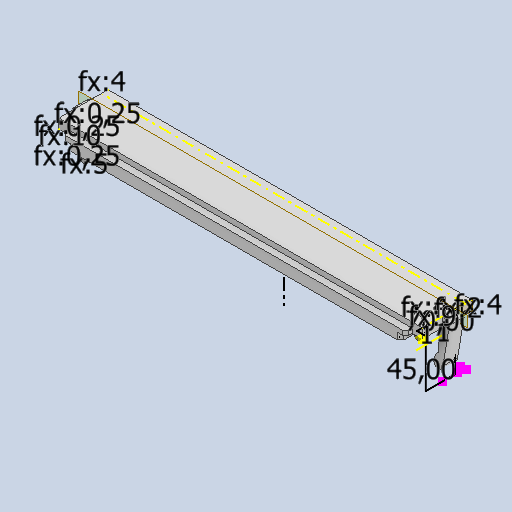
# Autodesk Inventor part: Generischer Gehäuse Deckel
Saved by Autodesk Inventor 2025.2 (Build 292293000, 293)
## iProperties
Created: 2025-11-01
Part Number: Generischer Gehäuse Deckel
Material: Generisch
Document SubType Name: Modeling
Designer: leowa
Density: 1 g/cm^3
Appearance: Vorgabe
Author: leowa
Autodesk Inventor part; units mm, degrees
ref_plane "YZ Plane" through (0, 0, 0) normal (1, 0, 0) x (0, 1, 0)
ref_plane "XZ Plane" through (0, 0, 0) normal (0, 1, 0) x (-1, 0, 0)
ref_plane "XY Plane" through (0, 0, 0) normal (0, 0, 1) x (1, 0, 0)
sketch "Skizze1" plane through (0, 0, 0) normal (0, 1, 0) x (-1, 0, 0)
  line L0 (0, 0) -> (108, 0)
  line L1 (108, 0) -> (108, -15)
  line L2 (108, -15) -> (0, -15)
  line L3 (0, -15) -> (0, 0)
  dimension "d0" = 108
  dimension "d1" = 15
  constraints: 8 end point, 2 parallel, 1 horizontal, 1 perpendicular
  measures "d0" distance of L1.end L2.end
  measures "d1" distance of L2.end L0.start
extrude "Extrusion1" add sketch "Skizze1" along normal blind 3
sketch "Skizze2" plane through (0, 0, 0) normal (0, -1, 0) x (1, 0, 0)
  line L0 (-108, 0) -> (0, 0) projected
  line L1 (-106.35, 0) -> (-1.65, 0)
  line L2 (-1.65, 0) -> (-1.65, 2)
  line L3 (-1.65, 2) -> (-106.35, 2)
  line L4 (-106.35, 2) -> (-106.35, 0)
  line L5 (-108, -15) -> (-108, 0) projected
  line L6 (0, -15) -> (-108, -15) projected
  line L7 (-54, -15) -> (-54, 78)
  point P0 (-54, 0)
  point P1 (-54, 2)
  dimension "d4" = 1.65
  dimension "d5" = 2
  constraints: 10 end point, 2 parallel, 1 horizontal, 1 midpoint, 1 perpendicular, 1 point on line, 1 vertical, 1 other
  measures "d4" distance between parallel lines of L4 L5
  measures "d5" distance between parallel lines of L0 L3
extrude "Extrusion2" add sketch "Skizze2" against normal blind 1.35 contours L4 L3 L7 L0 | L7 L3 L2 L0
sketch "Skizze3" plane through (0, 0, 0) normal (0, -1, 0) x (1, 0, 0)
  line L0 (0, -15) -> (-108, -15) projected
  line L1 (-106.65, -15) -> (-1.35, -15)
  line L2 (-1.35, -15) -> (-1.35, -13)
  line L3 (-1.35, -13) -> (-106.65, -13)
  line L4 (-106.65, -13) -> (-106.65, -15)
  line L5 (-54, -15) -> (-54, 54)
  line L6 (-108, -15) -> (-108, 0) projected
  point P0 (0, 0)
  dimension "d8" = 1.35
  dimension "d9" = 2
  constraints: 10 end point, 2 parallel, 1 horizontal, 1 midpoint, 1 perpendicular, 1 point on line, 1 vertical, 1 other
  measures "d8" distance between parallel lines of L6 L4
  measures "d9" distance of L3.end L1.start
extrude "Extrusion3" cut sketch "Skizze3" against normal blind 1.65
ref_plane "Arbeitsebene1" through (0, 3, -10) normal (0, 0, -1) x (-1, 0, 0)
sketch "Skizze4" plane through (0, 0, 0) normal (0, -1, 0) x (1, 0, 0)
  line L0 (21.6, -10) -> (-129.6, -10) projected
  line L1 (-104.875, -10) -> (-3.125, -10)
  line L2 (-3.125, -10) -> (-3.125, -13)
  line L3 (-3.125, -13) -> (-104.875, -13)
  line L4 (-104.875, -13) -> (-104.875, -10)
  line L5 (-106.65, -13) -> (-1.35, -13) projected
  line L6 (-1.35, -13) -> (-1.35, -15) projected
  line L7 (0, -15) -> (-108, -15) projected
  line L8 (-54, -15) -> (-54, 34)
  point P0 (0, 0)
  point P1 (-3.125, -10)
  dimension "d36" = 101.75
  constraints: 10 end point, 2 parallel, 1 collinear, 1 horizontal, 1 midpoint, 1 perpendicular, 1 point on line, 1 vertical, 1 other
  measures "d36" distance of L2.end L3.end
extrude "Extrusion4" add sketch "Skizze4" along normal blind 2 contours L2 L3 L8 L0 | L8 L3 L4 L0
sketch "Skizze5" plane through (0, 0, 0) normal (0, -1, 0) x (1, 0, 0)
  line L0 (-3.125, -8.02) -> (-104.875, -8.02)
  line L1 (-104.875, -8.02) -> (-104.875, 2)
  line L2 (-104.875, 2) -> (-3.125, 2)
  line L3 (-3.125, 2) -> (-3.125, -8.02)
  line L4 (-3.125, -10) -> (-104.875, -10) projected
  line L5 (-104.875, -10) -> (-104.875, -13) projected
  line L6 (-3.125, -13) -> (-3.125, -10) projected
  line L7 (-1.65, 2) -> (-106.35, 2) projected
  point P0 (0, 0)
  dimension "d16" = 1.98
  constraints: 8 end point, 3 collinear, 2 parallel, 1 horizontal, 1 perpendicular
  measures "d16" distance between parallel lines of L4 L0
extrude "Extrusion5" add sketch "Skizze5" along normal up to surface (2 mm away)
sketch "Skizze6" plane through (-108, 0, -15) normal (-1, 0, 0) x (0, 0, 1)
  line L0 (15, 3) -> (0, 3) projected
  line L1 (0, 3) -> (15, 3)
  line L2 (15, 3) -> (15, 0)
  line L3 (15, 0) -> (0, 0)
  line L4 (0, 0) -> (0, 3)
  constraints: 8 end point, 2 parallel, 1 horizontal, 1 perpendicular
extrude "Extrusion6" add sketch "Skizze6" along normal blind 1.5
sketch "Skizze9" plane through (0, 0, 0) normal (1, 0, 0) x (0, 0, -1)
  line L0 (0, 0) -> (15, 0) projected
  line L1 (15, 0) -> (15, 3) projected
  line L2 (0, 3) -> (15, 3) projected
  line L3 (0, 0) -> (0, 3) projected
extrude "Extrusion9" add sketch "Skizze9" along normal blind 1.5
sketch "Skizze7" plane through (-109.5, 0, -15) normal (-1, 0, 0) x (0, 0, 1)
  line L0 (15, 0) -> (0, 0) projected
  line L1 (4, 0) -> (9, 0) construction
  line L2 (9, 0) -> (9, -10) construction
  line L3 (9, -10) -> (4, -10) construction
  line L4 (4, -10) -> (4, 0) construction
  line L5 (0, 3) -> (0, 0) projected
  line L6 (4.25, 0) -> (8.75, 0)
  line L7 (8.75, 0) -> (8.75, -10.25)
  line L8 (8.75, -10.25) -> (4.25, -10.25)
  line L9 (4.25, -10.25) -> (4.25, 0)
  point P0 (9, 0)
  point P1 (8.75, 0)
  point P2 (4.25, 0)
  dimension "d22" = 4
  dimension "d23" = 5
  dimension "d24" = 10
  dimension "d37" = 0.25
  dimension "d38" = 0.25
  dimension "d39" = 0.25
  constraints: 16 end point, 4 parallel, 2 horizontal, 2 perpendicular, 2 point on line
  measures "d22" distance between parallel lines of L4 L5
  measures "d23" distance of L2.end L3.end
  measures "d24" distance of L1.end L2.end
  measures "d37" distance between parallel lines of L4 L9
  measures "d38" distance between parallel lines of L2 L7
  measures "d39" distance between parallel lines of L3 L8
extrude "Extrusion7" add sketch "Skizze7" against normal blind 1.25
extrude "Extrusion11" add sketch "Skizze7" along normal blind 1.25 from surface at -111
sketch "Skizze8" plane through (-109.5, -10, -6.25) normal (0, 0, 1) x (1, 0, 0)
  line L0 (0, 13) -> (111, 13) projected
  line L1 (55.5, 13) -> (55.5, -32)
  line L2 (0, -0.25) -> (0, 10) projected
  line L3 (0, -0.25) -> (1.25, -0.25) projected
  line L4 (1.25, 10) -> (1.25, -0.25) projected
  line L5 (0, 10) -> (1.25, 10) projected
  line L6 (0, -0.25) -> (0, 10) projected
  line L7 (1.25, 10) -> (1.25, -0.25) projected
  line L8 (111, -0.25) -> (111, 10) projected
  arc A0 (2.75, -0.25) -> (1.25, 2.8725) centre (-1.25, -0.25) ccw
  arc A1 (0, -0.25) -> (2.75, -0.25) centre (1.375, -0.25) ccw
  line L9 (0, -0.25) -> (1.25, -0.25)
  line L10 (1.25, 2.8725) -> (0, 2.8725)
  line L11 (0, -0.25) -> (0, 2.8725)
  line L12 (111, -0.25) -> (109.75, -0.25)
  arc A2 (109.75, 2.8725) -> (108.25, -0.25) centre (112.25, -0.25) ccw
  arc A3 (108.25, -0.25) -> (111, -0.25) centre (109.625, -0.25) ccw
  line L13 (111, -0.25) -> (109.75, -0.25)
  line L14 (109.75, 2.8725) -> (111, 2.8725)
  line L15 (111, -0.25) -> (111, 2.8725)
  point P0 (1.25, -4.25)
  point P1 (0, 2.8725)
  dimension "d76" = 4
  dimension "d77" = 1.5
  constraints: 16 end point, 8 point on circle, 7 point on line, 7 symmetric about line, 4 centre point, 2 collinear, 2 tangent, 1 midpoint, 1 perpendicular, 1 vertical, 2 other
  measures "d76" radius of A0
  measures "d77" distance from line of A0.start L4
extrude "Extrusion8" add sketch "Skizze8" against normal up to surface (4.5 mm away) contours L2 L10 L4 L3 | L3 L4 A0 A1 | A3 A2 L14 L8
sketch "Skizze11" plane through (0.25, 0, -6.25) normal (0, 0, 1) x (1, 0, 0)
  line L0 (1.25, 3) -> (-109.75, 3) projected
  line L1 (-54.25, 3) -> (-54.25, -19)
  line L2 (-109.75, 3) -> (1.25, 3)
  arc A0 (-1.5, -10.25) -> (1.25, -10.25) centre (-0.125, -10.25) ccw projected
  line L3 (1.25, -10.25) -> (3.25, 1.5)
  line L4 (3.25, 1.5) -> (1.25, 3)
  line L5 (1.25, 3) -> (1.25, 0) projected
  line L6 (1.25, 1.5) -> (5.25, 1.5) construction
  line L7 (1.25, -10.25) -> (1.25, 3) construction
  line L8 (1.25, -10.25) -> (1.25, 0) construction
  line L9 (-109.75, -10.25) -> (-111.75, 1.5)
  line L10 (-111.75, 1.5) -> (-109.75, 3)
  line L11 (-109.75, 3) -> (-109.75, 0)
  line L12 (-109.75, -10.25) -> (-109.75, 3) construction
  line L13 (-109.75, -10.25) -> (-109.75, 0) construction
  line L14 (1.25, -10.25) -> (1.25, 3)
  line L15 (-109.75, 0) -> (-109.75, 3) projected
  line L16 (-109.75, -10.25) -> (-109.75, 3)
  point P0 (-109.75, 1.5)
  point P1 (-109.75, 0)
  point P2 (1.25, 0)
  dimension "d78" = 2
  constraints: 26 end point, 8 symmetric about line, 3 collinear, 3 midpoint, 1 horizontal, 1 vertical
  measures "d78" distance of L3.end L6.start
extrude "Extrusion12" add sketch "Skizze11" against normal up to surface (4.5 mm away)
sketch "Skizze12" plane through (-1.35, 1.65, -13) normal (0, 0, -1) x (-1, 0, 0)
  line L0 (1.775, -1.65) -> (1.775, -3.65) projected
  line L1 (1.775, -3.65) -> (3.2309, -7.65)
  line L2 (3.2309, -7.65) -> (4.2309, -7.65)
  line L3 (4.2309, -7.65) -> (5.6868, -3.65)
  line L4 (103.525, -3.65) -> (1.775, -3.65) projected
  line L5 (-1.6, -15.9) -> (-3.35, -15.9) projected
  line L6 (-2.85, 1.35) -> (108.15, 1.35) projected
  line L7 (52.65, 1.35) -> (52.65, -27)
  line L8 (1.775, -3.65) -> (5.6868, -3.65)
  line L9 (103.525, -3.65) -> (102.0691, -7.65)
  line L10 (102.0691, -7.65) -> (101.0691, -7.65)
  line L11 (101.0691, -7.65) -> (99.6132, -3.65)
  line L12 (103.525, -3.65) -> (99.6132, -3.65)
  point P0 (-1.35, -1.65)
  dimension "d52" = 70
  dimension "d53" = 1
  dimension "d55" = 4
  constraints: 18 end point, 3 symmetric about line, 1 collinear, 1 equal length, 1 midpoint, 1 perpendicular, 1 point on line, 1 vertical
  measures "d52" angle of L4 L1
  measures "d53" distance of L1.end L2.end
  measures "d55" distance between parallel lines of L4 L2
extrude "Extrusion13" add sketch "Skizze12" against normal up to surface (3 mm away)
extrude "Extrusion14" add sketch "Skizze12" against normal blind 3 from surface at -4.98
chamfer "Fasen2" distance 1 angle 45 4 edges at (-106.35, 0.675, 2) (-104.875, -1, 2) (-1.65, 0.675, 2) (-3.125, -1, 2)
ref_plane "Arbeitsebene2" through (1.5, 0, 0) normal (1, 0, 0) x (0, 0, -1)
sketch "Skizze13" plane through (1.5, 0, 0) normal (1, 0, 0) x (0, 0, -1)
  point P0 (0, 0)
sketch "Skizze14" plane through (1.5, 0, 0) normal (1, 0, 0) x (0, 0, -1)
  line L0 (-2, -2) -> (-1, -2) projected
  line L1 (-1, -2) -> (-2, -2) projected
  line L2 (5.02, -2) -> (-1, -2) projected
  line L3 (5.02, -2) -> (8.02, -2) projected
  line L4 (8.02, -2) -> (5.02, -2) projected
  line L5 (-1, -2) -> (5.02, -2) projected
  line L6 (10, -6) -> (10, -2) projected
  line L7 (10, -2) -> (10, -6) projected
  line L8 (10, 0) -> (10, -2) projected
  line L9 (10, 0) -> (10, -2) projected
  line L10 (10, -6) -> (10, -2) projected
  line L11 (10, -2) -> (10, -6) projected
  line L12 (0, 3) -> (6.25, 3) projected
  line L13 (6.25, 3) -> (0, 3) projected
  line L14 (10.75, 3) -> (6.25, 3) projected
  line L15 (15, 3) -> (10.75, 3) projected
  line L16 (10.75, 3) -> (15, 3) projected
  line L17 (6.25, 3) -> (10.75, 3) projected
  line L18 (10, -14.25) -> (1, -14.25)
  line L19 (1, -14.25) -> (1, 3)
  line L20 (1, 3) -> (10, 3)
  line L21 (10, 3) -> (10, -14.25)
  line L22 (10, 3) -> (12, 3)
  line L23 (12, 3) -> (12, -1)
  line L24 (12, -1) -> (10, -1)
  line L25 (10, -1) -> (10, 3)
  line L26 (1, 0.35) -> (-1.65, 3)
  line L27 (-1.65, 3) -> (1, 3)
  line L28 (-1, 1.35) -> (-2, 1.35) projected
  line L29 (-1, 1.35) -> (0, 1.35) projected
  line L30 (0, 1.35) -> (-1, 1.35) projected
  line L31 (-2, 1.35) -> (-1, 1.35) projected
  line L32 (0, 1.35) -> (1, 1.35) construction
  line L33 (6.25, -14.25) -> (10.75, -14.25) projected
  line L34 (6.25, -14.25) -> (10.75, -14.25) projected
  line L35 (6.25, -14.25) -> (10.75, -14.25) projected
  point P0 (0, 0)
  dimension "d64" = 9
  dimension "d65" = 2
  dimension "d66" = 4
  dimension "d67" = 45
  dimension "d69" = 1
  constraints: 22 end point, 4 parallel, 3 collinear, 3 horizontal, 3 perpendicular, 2 point on line
  measures "d64" distance between parallel lines of L19 L21
  measures "d65" distance of L23.end L24.end
  measures "d66" distance of L22.end L23.end
  measures "d67" angle of L19 L26
  measures "d69" distance of L26.start L32.end
equation "\"d0\" = Modul_Grundflächenlänge + 2 * Wandstärke"
equation "\"d1\" = Generische_Modulbreite"
equation "\"d2\" = Deckelstärke"
equation "\"d4\" = 0.55 * Basisstärke"
equation "\"d5\" = Modulüberlappung"
equation "\"d6\" = 0.45 * Deckelstärke"
equation "\"d8\" = 0.45 * Basisstärke"
equation "\"d9\" = Modulüberlappung"
equation "\"d10\" = 0.55 * Deckelstärke"
equation "\"d36\" = Modul_Grundflächenlänge - 0.5 * Stecktoleranz"
equation "\"d14\" = Deckel_Verstärkung"
equation "\"d16\" = 1.1 * Platinendicke"
equation "\"d20\" = Deckel_Klipperstärke"
equation "\"d31\" = Deckel_Klipperstärke"
equation "\"d22\" = Deckel_Klipperposition"
equation "\"d23\" = Deckel_Klippbreite"
equation "\"d24\" = Deckel_Klipplänge"
equation "\"d37\" = 0.5 * Stecktoleranz"
equation "\"d38\" = 0.5 * Stecktoleranz"
equation "\"d39\" = 0.5 * Stecktoleranz"
equation "\"d25\" = Deckel_Klipperstärke - 0.5 * Stecktoleranz"
equation "\"d40\" = Deckel_Klipperstärke - 0.5 * Stecktoleranz"
equation "\"d76\" = Deckelklipper_Radius"
equation "\"d77\" = Deckel_Klipptiefe"
equation "\"d55\" = Deckel_Einrastführungslänge"
equation "\"d64\" = Steckverbinder_Lochtiefe"
equation "\"d65\" = Steckverbinder_Absatzbreite"
equation "\"d66\" = Steckverbinder_Absatztiefe"
equation "\"Wandstärke\" = 3"
equation "\"Basisstärke\" = 3"
equation "\"Modulüberlappung\" = 2"
equation "\"Platinendicke\" = 1.8"
equation "\"Deckelstärke\" = 3"
equation "\"Seitenwand_Höhe\" = 39"
equation "\"Platinenposition\" = 5"
equation "\"d12\" = -Platinenposition"
equation "\"Deckel_Klippbreite\" = 5"
equation "\"Deckel_Klipplänge\" = 10"
equation "\"Deckel_Klipperposition\" = 4"
equation "\"Deckel_Klipperstärke\" = 1.5"
equation "\"Deckel_Klipptiefe\" = 1.5"
equation "\"Modul_Klipptiefe\" = 1.5"
equation "\"Modul_Klipperstärke\" = 1.5"
equation "\"Modul_Klipperposition\" = 7"
equation "\"Modul_Klipplänge\" = 8"
equation "\"Lüftungsraster\" = 2"
equation "\"Dings\" = 2"
equation "\"Modul_Grundflächenlänge\" = 102"
equation "\"Relais_Modulbreite\" = 28"
equation "\"Generische_Modulbreite\" = 15"
equation "\"Steckverbinderabsatztiefe\" = 4"
equation "\"Steckverbinder_Absatztiefe\" = 4"
equation "\"Steckverbinder_Absatzbreite\" = 2"
equation "\"Steckverbinder_Lochtiefe\" = 9"
equation "\"Steckverbinder_Fasenbreite\" = 1"
equation "\"Hauptmodul_Klipperabstand\" = 15"
equation "\"Stecktoleranz\" = 0.5"
equation "\"Rahmen_Durchbiegungsstopp\" = 5"
equation "\"Deckel_Einrastführungslänge\" = 4"
equation "\"Deckel_Verstärkung\" = 2"
equation "\"Deckelklipper_Radius\" = 4"
equation "\"Montage_Langloch\" = 5"
equation "\"Montage_Modulbreite\" = 15"
equation "\"Deckklipper_Kantenverrundung\" = 1"
equation "\"Montage_Bohrung\" = 4.5"
equation "\"Hauptmodul_Stufenposition\" = 53"
equation "\"Hauptmodulbreite\" = 28"
equation "\"Hauptmodul_Platinenhöhe_lang\" = 61"
equation "\"Hauptmodul_Platinenhöhe_kurz\" = 48"
equation "\"Generische_Platinenhöhe\" = 38"
equation "\"Modul_Klipperradius\" = 2"
equation "\"Modul_Klipper_Kantenverrundung\" = 1"
equation "\"Test_Schnittabstand\" = 5"
equation "\"Montage_Schwalbenschwanz_Winkel\" = 30deg"
equation "\"Montage_Schwalbenschwanz_Länge\" = 3"
equation "\"Hauptmodul_Deckel_Einschubtiefe\" = 2"
